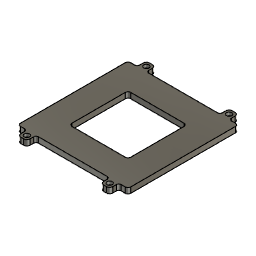
bottom_mount (Autodesk Fusion 360 design; units mm, degrees)
Autodesk Fusion 360 part; units mm, degrees
sketch "Sketch1" plane through (0, 0, 0) normal (0, 0, 1) x (1, 0, 0)
  line L0 (60, -60) -> (-60, -60)
  line L1 (-60, -60) -> (-60, 60)
  line L2 (-60, 60) -> (60, 60)
  line L3 (60, 60) -> (60, -60)
  line L4 (60, -60) -> (-60, 60) construction
  line L5 (-60, -60) -> (60, 60) construction
  dimension "d4" = 120
  dimension "d5" = 120
  constraint perpendicular L0 L1
  constraint parallel L0 L2
  constraint parallel L1 L3
  constraint horizontal L0
  constraint coincident L4 origin
  constraint coincident L5 origin
  measures "d4" distance of L1.end L2.end
  measures "d5" distance of L0.end L1.end
extrude "Extrude1" add sketch "Sketch1" along normal blind 6
sketch "Sketch6" plane through (0, 0, 6) normal (0, 0, 1) x (-1, 0, 0)
  line L0 (-60, -60) -> (60, -60)
  line L1 (60, -60) -> (60, 60)
  line L2 (60, 60) -> (-60, 60)
  line L3 (-60, 60) -> (-60, -60)
sketch "Sketch7" plane through (0, 0, 6) normal (0, 0, 1) x (-1, 0, 0)
  line L0 (-60, -60) -> (60, -60)
  line L1 (60, -60) -> (60, 60)
  line L2 (60, 60) -> (-60, 60)
  line L3 (-60, 60) -> (-60, -60)
  line L4 (50, 60) -> (40, 60)
  line L5 (40, 60) -> (40, 70)
  line L6 (40, 70) -> (50, 70)
  line L7 (50, 70) -> (50, 60)
  circle A0 centre (45, 65) radius 1.625
  line L8 (0, -80) -> (0, 80) construction
  line L9 (75, 0) -> (-75, 0) construction
  circle A1 centre (-45, 65) radius 1.625
  line L10 (-50, 60) -> (-40, 60)
  line L11 (-40, 70) -> (-50, 70)
  line L12 (-40, 60) -> (-40, 70)
  line L13 (-50, 70) -> (-50, 60)
  line L14 (40, -70) -> (50, -70)
  line L15 (0, 80) -> (0, -80) construction
  line L16 (-40, -70) -> (-50, -70)
  line L17 (50, -60) -> (40, -60)
  circle A2 centre (-45, -65) radius 1.625
  line L18 (40, -60) -> (40, -70)
  circle A3 centre (45, -65) radius 1.625
  line L19 (50, -70) -> (50, -60)
  line L20 (-40, -60) -> (-40, -70)
  line L21 (-50, -70) -> (-50, -60)
  dimension "d78" = 10
  dimension "d79" = 10
  dimension "d80" = 10
  dimension "d81" = 3.25
  dimension "d83" = 5
  dimension "d84" = 5
  constraint horizontal L4
  constraint vertical L5
  constraint horizontal L6
  constraint vertical L7
  constraint coincident L2 L4.start
  constraint parallel L3 L8
  constraint perpendicular L3 L9
  constraint symmetric L4.start L8 L10.start
  constraint symmetric L4.end L8 L10.end
  constraint symmetric L5.end L8 L11.start
  constraint symmetric L6.end L8 L11.end
  constraint symmetric A0 L8 A1
  constraint symmetric L4.start L9 L17.start
  constraint symmetric L4.end L9 L17.end
  constraint symmetric L5.end L9 L14.start
  constraint symmetric L6.end L9 L14.end
  constraint symmetric A0 L9 A3
  constraint symmetric L8.start L9 L8.end
  constraint symmetric L8.end L9 L8.start
  constraint symmetric L9 L10.end L20.start
  constraint symmetric L9 L10.start L21.end
  constraint symmetric L9 L11.end L16.end
  constraint symmetric L9 L11.start L16.start
  constraint symmetric L9 A1 A2
  measures "d78" distance of L4.start L4.end
  measures "d79" distance of L4.start L6.end
  measures "d80" distance of L1 L7
  measures "d81" diameter of A0
  measures "d83" distance of L6 A0.centre
  measures "d84" distance of L5 A0.centre
extrude "Extrude7" add sketch "Sketch7" against normal up to surface (6 mm away) contours L0 L16 L20 L21 | L2 L10 L11 L12 L13 | L0 L14 L17 L18 L19 | L2 L4 L5 L6 L7
fillet "Fillet1" radius 3.5 2 edges at (-50, -70, 3) (-40, -70, 3)
fillet "Fillet2" radius 3.5 2 edges at (40, -70, 3) (50, -70, 3)
fillet "Fillet3" radius 3.5 2 edges at (-40, 70, 3) (-50, 70, 3)
fillet "Fillet4" radius 3.5 2 edges at (40, 70, 3) (50, 70, 3)
fillet "Fillet5" radius 2.5 8 edges at (50, 60, 3) (40, 60, 3) (-40, 60, 3) (-50, 60, 3) (-50, -60, 3) (50, -60, 3) (-40, -60, 3) (40, -60, 3)
fillet "Fillet6" radius 3 4 edges at (-60, 60, 3) (-60, -60, 3) (60, -60, 3) (60, 60, 3)
sketch "Sketch8" plane through (0, 0, 6) normal (0, 0, 1) x (-1, 0, 0)
  circle A0 centre (45, -65) radius 1.625
  circle A1 centre (45, 65) radius 1.625
  circle A2 centre (-45, -65) radius 1.625
  circle A3 centre (-45, 65) radius 1.625
  arc A4 (-60, -57) -> (-57, -60) centre (-57, -57) ccw
  line L0 (-57, -60) -> (-52.5, -60)
  arc A5 (-50, -62.5) -> (-52.5, -60) centre (-52.5, -62.5) ccw
  line L1 (-50, -62.5) -> (-50, -66.5)
  arc A6 (-50, -66.5) -> (-46.5, -70) centre (-46.5, -66.5) ccw
  line L2 (-46.5, -70) -> (-43.5, -70)
  arc A7 (-43.5, -70) -> (-40, -66.5) centre (-43.5, -66.5) ccw
  line L3 (-40, -66.5) -> (-40, -62.5)
  arc A8 (-37.5, -60) -> (-40, -62.5) centre (-37.5, -62.5) ccw
  line L4 (-37.5, -60) -> (37.5, -60)
  arc A9 (40, -62.5) -> (37.5, -60) centre (37.5, -62.5) ccw
  line L5 (40, -62.5) -> (40, -66.5)
  arc A10 (40, -66.5) -> (43.5, -70) centre (43.5, -66.5) ccw
  line L6 (43.5, -70) -> (46.5, -70)
  arc A11 (46.5, -70) -> (50, -66.5) centre (46.5, -66.5) ccw
  line L7 (50, -66.5) -> (50, -62.5)
  arc A12 (52.5, -60) -> (50, -62.5) centre (52.5, -62.5) ccw
  line L8 (52.5, -60) -> (57, -60)
  arc A13 (57, -60) -> (60, -57) centre (57, -57) ccw
  line L9 (60, -57) -> (60, 57)
  arc A14 (60, 57) -> (57, 60) centre (57, 57) ccw
  line L10 (57, 60) -> (52.5, 60)
  arc A15 (50, 62.5) -> (52.5, 60) centre (52.5, 62.5) ccw
  line L11 (50, 62.5) -> (50, 66.5)
  arc A16 (50, 66.5) -> (46.5, 70) centre (46.5, 66.5) ccw
  line L12 (46.5, 70) -> (43.5, 70)
  arc A17 (43.5, 70) -> (40, 66.5) centre (43.5, 66.5) ccw
  line L13 (40, 66.5) -> (40, 62.5)
  arc A18 (37.5, 60) -> (40, 62.5) centre (37.5, 62.5) ccw
  line L14 (37.5, 60) -> (-37.5, 60)
  arc A19 (-40, 62.5) -> (-37.5, 60) centre (-37.5, 62.5) ccw
  line L15 (-40, 62.5) -> (-40, 66.5)
  arc A20 (-40, 66.5) -> (-43.5, 70) centre (-43.5, 66.5) ccw
  line L16 (-43.5, 70) -> (-46.5, 70)
  arc A21 (-46.5, 70) -> (-50, 66.5) centre (-46.5, 66.5) ccw
  line L17 (-50, 66.5) -> (-50, 62.5)
  arc A22 (-52.5, 60) -> (-50, 62.5) centre (-52.5, 62.5) ccw
  line L18 (-52.5, 60) -> (-57, 60)
  arc A23 (-57, 60) -> (-60, 57) centre (-57, 57) ccw
  line L19 (-60, 57) -> (-60, -57)
  circle A24 centre (45, 65) radius 2.875
  dimension "d98" = 5.75
  constraint concentric A1 A24
  measures "d98" diameter of A24
extrude "Extrude8" cut sketch "Sketch8" against normal blind 3.5 contours A24
sketch "Sketch9" plane through (0, 0, 6) normal (0, 0, 1) x (-1, 0, 0)
  circle A0 centre (45, 65) radius 2.875
  circle A1 centre (45, -65) radius 1.625
  circle A2 centre (-45, -65) radius 1.625
  circle A3 centre (-45, 65) radius 1.625
  arc A4 (-60, -57) -> (-57, -60) centre (-57, -57) ccw
  line L0 (-57, -60) -> (-52.5, -60)
  arc A5 (-50, -62.5) -> (-52.5, -60) centre (-52.5, -62.5) ccw
  line L1 (-50, -62.5) -> (-50, -66.5)
  arc A6 (-50, -66.5) -> (-46.5, -70) centre (-46.5, -66.5) ccw
  line L2 (-46.5, -70) -> (-43.5, -70)
  arc A7 (-43.5, -70) -> (-40, -66.5) centre (-43.5, -66.5) ccw
  line L3 (-40, -66.5) -> (-40, -62.5)
  arc A8 (-37.5, -60) -> (-40, -62.5) centre (-37.5, -62.5) ccw
  line L4 (-37.5, -60) -> (37.5, -60)
  arc A9 (40, -62.5) -> (37.5, -60) centre (37.5, -62.5) ccw
  line L5 (40, -62.5) -> (40, -66.5)
  arc A10 (40, -66.5) -> (43.5, -70) centre (43.5, -66.5) ccw
  line L6 (43.5, -70) -> (46.5, -70)
  arc A11 (46.5, -70) -> (50, -66.5) centre (46.5, -66.5) ccw
  line L7 (50, -66.5) -> (50, -62.5)
  arc A12 (52.5, -60) -> (50, -62.5) centre (52.5, -62.5) ccw
  line L8 (52.5, -60) -> (57, -60)
  arc A13 (57, -60) -> (60, -57) centre (57, -57) ccw
  line L9 (60, -57) -> (60, 57)
  arc A14 (60, 57) -> (57, 60) centre (57, 57) ccw
  line L10 (57, 60) -> (52.5, 60)
  arc A15 (50, 62.5) -> (52.5, 60) centre (52.5, 62.5) ccw
  line L11 (50, 62.5) -> (50, 66.5)
  arc A16 (50, 66.5) -> (46.5, 70) centre (46.5, 66.5) ccw
  line L12 (46.5, 70) -> (43.5, 70)
  arc A17 (43.5, 70) -> (40, 66.5) centre (43.5, 66.5) ccw
  line L13 (40, 66.5) -> (40, 62.5)
  arc A18 (37.5, 60) -> (40, 62.5) centre (37.5, 62.5) ccw
  line L14 (37.5, 60) -> (-37.5, 60)
  arc A19 (-40, 62.5) -> (-37.5, 60) centre (-37.5, 62.5) ccw
  line L15 (-40, 62.5) -> (-40, 66.5)
  arc A20 (-40, 66.5) -> (-43.5, 70) centre (-43.5, 66.5) ccw
  line L16 (-43.5, 70) -> (-46.5, 70)
  arc A21 (-46.5, 70) -> (-50, 66.5) centre (-46.5, 66.5) ccw
  line L17 (-50, 66.5) -> (-50, 62.5)
  arc A22 (-52.5, 60) -> (-50, 62.5) centre (-52.5, 62.5) ccw
  line L18 (-52.5, 60) -> (-57, 60)
  arc A23 (-57, 60) -> (-60, 57) centre (-57, 57) ccw
  line L19 (-60, 57) -> (-60, -57)
  circle A24 centre (-45, 65) radius 2.875
  circle A25 centre (-45, -65) radius 2.875
  circle A26 centre (45, -65) radius 2.875
  dimension "d101" = 5.75
  dimension "d102" = 5.75
  dimension "d103" = 5.75
  constraint concentric A3 A24
  constraint concentric A2 A25
  constraint concentric A1 A26
  measures "d101" diameter of A24
  measures "d102" diameter of A25
  measures "d103" diameter of A26
extrude "Extrude9" cut sketch "Sketch9" against normal blind 3.5 contours A24 | A25 | A26
sketch "Sketch10" plane through (0, 0, 6) normal (0, 0, 1) x (-1, 0, 0)
  circle A0 centre (-45, 65) radius 2.875
  circle A1 centre (-45, -65) radius 2.875
  circle A2 centre (45, -65) radius 2.875
  circle A3 centre (45, 65) radius 2.875
  arc A4 (-60, -57) -> (-57, -60) centre (-57, -57) ccw
  line L0 (-57, -60) -> (-52.5, -60)
  arc A5 (-50, -62.5) -> (-52.5, -60) centre (-52.5, -62.5) ccw
  line L1 (-50, -62.5) -> (-50, -66.5)
  arc A6 (-50, -66.5) -> (-46.5, -70) centre (-46.5, -66.5) ccw
  line L2 (-46.5, -70) -> (-43.5, -70)
  arc A7 (-43.5, -70) -> (-40, -66.5) centre (-43.5, -66.5) ccw
  line L3 (-40, -66.5) -> (-40, -62.5)
  arc A8 (-37.5, -60) -> (-40, -62.5) centre (-37.5, -62.5) ccw
  line L4 (-37.5, -60) -> (37.5, -60)
  arc A9 (40, -62.5) -> (37.5, -60) centre (37.5, -62.5) ccw
  line L5 (40, -62.5) -> (40, -66.5)
  arc A10 (40, -66.5) -> (43.5, -70) centre (43.5, -66.5) ccw
  line L6 (43.5, -70) -> (46.5, -70)
  arc A11 (46.5, -70) -> (50, -66.5) centre (46.5, -66.5) ccw
  line L7 (50, -66.5) -> (50, -62.5)
  arc A12 (52.5, -60) -> (50, -62.5) centre (52.5, -62.5) ccw
  line L8 (52.5, -60) -> (57, -60)
  arc A13 (57, -60) -> (60, -57) centre (57, -57) ccw
  line L9 (60, -57) -> (60, 57)
  arc A14 (60, 57) -> (57, 60) centre (57, 57) ccw
  line L10 (57, 60) -> (52.5, 60)
  arc A15 (50, 62.5) -> (52.5, 60) centre (52.5, 62.5) ccw
  line L11 (50, 62.5) -> (50, 66.5)
  arc A16 (50, 66.5) -> (46.5, 70) centre (46.5, 66.5) ccw
  line L12 (46.5, 70) -> (43.5, 70)
  arc A17 (43.5, 70) -> (40, 66.5) centre (43.5, 66.5) ccw
  line L13 (40, 66.5) -> (40, 62.5)
  arc A18 (37.5, 60) -> (40, 62.5) centre (37.5, 62.5) ccw
  line L14 (37.5, 60) -> (-37.5, 60)
  arc A19 (-40, 62.5) -> (-37.5, 60) centre (-37.5, 62.5) ccw
  line L15 (-40, 62.5) -> (-40, 66.5)
  arc A20 (-40, 66.5) -> (-43.5, 70) centre (-43.5, 66.5) ccw
  line L16 (-43.5, 70) -> (-46.5, 70)
  arc A21 (-46.5, 70) -> (-50, 66.5) centre (-46.5, 66.5) ccw
  line L17 (-50, 66.5) -> (-50, 62.5)
  arc A22 (-52.5, 60) -> (-50, 62.5) centre (-52.5, 62.5) ccw
  line L18 (-52.5, 60) -> (-57, 60)
  arc A23 (-57, 60) -> (-60, 57) centre (-57, 57) ccw
  line L19 (-60, 57) -> (-60, -57)
  line L20 (-32, 32) -> (32, 32)
  line L21 (32, 32) -> (32, -32)
  line L22 (32, -32) -> (-32, -32)
  line L23 (-32, -32) -> (-32, 32)
  line L24 (-32, 32) -> (32, -32) construction
  line L25 (32, 32) -> (-32, -32) construction
  dimension "d108" = 64
  dimension "d109" = 64
  constraint perpendicular L20 L21
  constraint parallel L20 L22
  constraint parallel L21 L23
  constraint horizontal L20
  constraint coincident L24 origin
  constraint coincident L25 origin
  measures "d108" distance of L21.end L22.end
  measures "d109" distance of L20.end L21.end
extrude "Extrude10" cut sketch "Sketch10" against normal up to surface (6 mm away) contours L20 L21 L22 L23
fillet "Fillet7" radius 3 4 edges at (32, 32, 3) (32, -32, 3) (-32, 32, 3) (-32, -32, 3)
equation "base_width = 120 mm"
equation "base_length = 120 mm"
equation "base_thickness = 6 mm"
equation "d4 = base_width"
equation "d5 = base_length"
equation "d6 = base_thickness"
equation "fan_mount_hole_long_edge_offset = 18 mm"
equation "fan_bottom_mount_hole_head_countersink = 3.5 mm"
equation "fan_bottom_mount_hole_diameter = 3.25 mm"
equation "fan_bottom_mount_hole_head_diameter = 5.75 mm"
equation "fan_bottom_mount_hole_slot_length = 4 mm"
equation "fan_mount_hole_short_edge_offset = 12.5 mm"
equation "pi_mount_width = 65.7 mm"
equation "pi_mount_length = 100.7 mm"
equation "pi_bottom_mount_hole_diameter = 3.25 mm"
equation "pi_bottom_mount_hole_head_countersink = 3.5 mm"
equation "pi_bottom_mount_hole_head_diameter = 5.75 mm"
equation "pi_bottom_mount_hole_slot_length = 8 mm"
equation "switch_width = 100 mm"
equation "switch_length = 98.5 mm"
equation "switch_lateral_support_length = 10 mm"
equation "switch_lateral_support_offset = 0.4 mm"
equation "switch_lateral_support_thickness = 1 mm"
equation "switch_lateral_support_width = 2 mm"
equation "base_bracket_width = 10 mm"
equation "base_bracket_edge_offset = 10 mm"
equation "base_bracket_hole_diameter = 3.25 mm"
equation "base_bracket_length = 10 mm"
equation "base_bracket_hole_edge_offset = 5 mm"
equation "d78 = base_bracket_width"
equation "d79 = base_bracket_length"
equation "d80 = base_bracket_edge_offset"
equation "d81 = base_bracket_hole_diameter"
equation "base_bracket_length_edge_offset = 5 mm"
equation "d83 = base_bracket_length_edge_offset"
equation "d84 = base_bracket_width / 2"
equation "base_bracket_outer_fillet = 3.5 mm"
equation "base_bracket_inner_fillet = 2.5 mm"
equation "d89 = base_bracket_outer_fillet"
equation "d90 = base_bracket_outer_fillet"
equation "d91 = base_bracket_outer_fillet"
equation "d92 = base_bracket_outer_fillet"
equation "d93 = base_bracket_inner_fillet"
equation "base_edge_fillet = 3 mm"
equation "d95 = base_edge_fillet"
equation "base_bracket_bottom_mount_hole_head_countersink = 3.5 mm"
equation "base_bracket_bottom_mount_hole_head_diameter = 5.75 mm"
equation "d98 = base_bracket_bottom_mount_hole_head_diameter"
equation "d99 = -base_bracket_bottom_mount_hole_head_countersink"
equation "d101 = base_bracket_bottom_mount_hole_head_diameter"
equation "d102 = base_bracket_bottom_mount_hole_head_diameter"
equation "d103 = base_bracket_bottom_mount_hole_head_diameter"
equation "d104 = -base_bracket_bottom_mount_hole_head_countersink"
equation "internal_hole_width = 64 mm"
equation "internal_hole_length = 64 mm"
equation "d108 = internal_hole_width"
equation "d109 = internal_hole_length"
equation "internal_hole_fillet = 3 mm"
equation "d113 = internal_hole_fillet"
